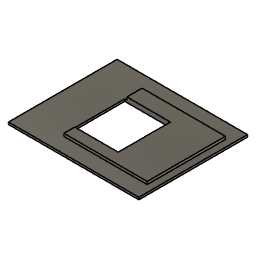
table_top v9 (Autodesk Fusion 360 design; units mm, degrees)
Autodesk Fusion 360 part; units mm, degrees
note: some values were not read from the file. Set by a fixed rule: which sketch regions a step uses.
sketch "Sketch1" plane through (0, 0, 0) normal (0, 0, 1) x (1, 0, 0)
  line L0 (0, 0) -> (152.4, 0)
  line L1 (152.4, 0) -> (152.4, 127)
  line L2 (152.4, 127) -> (0, 127)
  line L3 (0, 127) -> (0, 0)
  line L4 (46.99, 109.22) -> (144.399, 109.22)
  line L5 (144.399, 109.22) -> (144.399, 17.78)
  line L6 (144.399, 17.78) -> (46.99, 17.78)
  line L7 (46.99, 17.78) -> (46.99, 109.22)
  dimension "d1" = 152.4
  dimension "d2" = 127
  dimension "d3" = 97.409
  dimension "d4" = 91.44
  dimension "d5" = 46.99
  dimension "d6" = 17.78
  constraint horizontal L0
  constraint vertical L1
  constraint horizontal L2
  constraint vertical L3
  constraint coincident L0.start L3.end
  constraint horizontal L4
  constraint vertical L5
  constraint horizontal L6
  constraint vertical L7
  measures "d1" distance of L0.start L0.end
  measures "d2" distance of L0.start L2.end
  measures "d3" distance of L4.start L4.end
  measures "d4" distance of L4.start L6.end
  measures "d5" distance of L3 L7
  measures "d6" distance of L0 L6
extrude "Extrude1" add sketch "Sketch1" along normal blind 2.54 contours L0 L1 L2 L3 | L4 L5 L6 L7
extrude "Extrude2" add sketch "Sketch1" along normal blind 5.715 contours L4 L5 L6 L7
sketch "Sketch2" plane through (0, 0, 5.715) normal (0, 0, 1) x (-1, 0, 0)
  line L0 (-46.99, -17.78) -> (-144.399, -17.78)
  line L1 (-144.399, -17.78) -> (-144.399, -109.22)
  line L2 (-144.399, -109.22) -> (-46.99, -109.22)
  line L3 (-46.99, -109.22) -> (-46.99, -17.78)
  line L4 (-46.99, -91.44) -> (-97.79, -91.44)
  line L5 (-97.79, -91.44) -> (-97.79, -30.48)
  line L6 (-97.79, -30.48) -> (-46.99, -30.48)
  line L7 (-46.99, -25.4) -> (-46.99, -30.48)
  line L8 (-46.99, -91.44) -> (-44.45, -91.44)
  line L9 (-44.45, -91.44) -> (-44.45, -30.48)
  line L10 (-44.45, -30.48) -> (-46.99, -30.48)
  line L11 (-46.99, -30.48) -> (-46.99, -91.44)
  dimension "d11" = 60.96
  dimension "d12" = 17.78
  dimension "d15" = 50.8
  dimension "d19" = 2.54
  dimension "d20" = 60.96
  constraint horizontal L4
  constraint vertical L5
  constraint horizontal L6
  constraint coincident L3 L4.start
  constraint vertical L7
  constraint horizontal L8
  constraint vertical L9
  constraint horizontal L10
  constraint vertical L11
  measures "d11" distance of L4.start L6.end
  measures "d12" distance of L2 L4
  measures "d15" distance of L4.start L4.end
  measures "d19" distance of L4.start L8.end
  measures "d20" distance of L4.start L6.end
extrude "Extrude3" cut sketch "Sketch2" against normal blind 38.1 contours L3 L4 L5 L6 L11
extrude "Extrude4" cut sketch "Sketch2" against normal blind 60.96 contours L3 L8 L9 L10 L11
